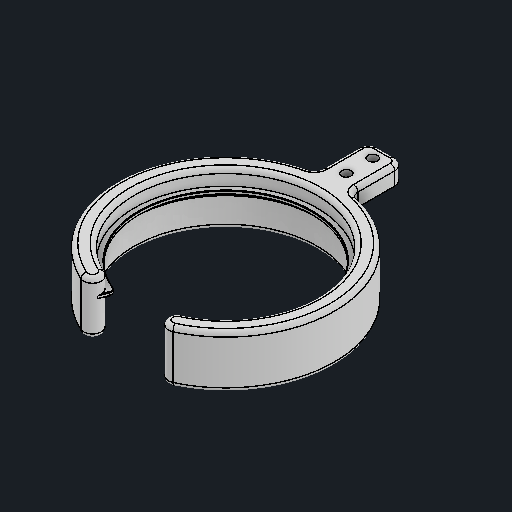
# Autodesk Inventor part: Can Clip
Saved by Autodesk Inventor 2026.2 (Build 302298000, 298)
## iProperties
Created: 2026-06-30
Part Number: Can Clip
Material: Generic
Document SubType Name: Modeling
Designer: JoshuaEah
Density: 1 g/cm^3
Appearance: Default
Author: JoshuaEah
Autodesk Inventor part; units mm, degrees
ref_plane "YZ Plane" through (0, 0, 0) normal (1, 0, 0) x (0, 1, 0)
ref_plane "XZ Plane" through (0, 0, 0) normal (0, 1, 0) x (-1, 0, 0)
ref_plane "XY Plane" through (0, 0, 0) normal (0, 0, 1) x (1, 0, 0)
sketch "Sketch1" plane through (0, 0, 0) normal (0, 1, 0) x (-1, 0, 0)
  circle A0 centre (0, 0) radius 33.02
  circle A1 centre (0, 0) radius 39.37
  line L0 (-10.642, 29.2385) -> (-13.4653, 36.9957)
  line L1 (0, 33.02) -> (0, -33.02)
  line L2 (10.642, 29.2385) -> (13.4653, 36.9957)
  line L3 (-6.35, -38.8545) -> (-6.35, -57.9045)
  line L4 (6.35, -38.8545) -> (6.35, -57.9045)
  line L5 (6.35, -57.9045) -> (-6.35, -57.9045)
  circle A2 centre (0, 0) radius 31.115
  circle A3 centre (0, -53.142) radius 1.5875
  line L6 (6.35, -48.3795) -> (-6.35, -48.3795) construction
  circle A4 centre (0, -43.617) radius 1.5875
  point P0 (13.4653, 36.9957)
  point P1 (11.2935, 31.0287)
  point P2 (-11.2935, 31.0287)
  point P3 (0, -31.115)
  point P4 (0, -48.3795)
  dimension "d11" = 62.23
  dimension "d0" = 66.04
  dimension "d1" = 6.35
  dimension "d2" = 20
  dimension "d5" = 12.7
  dimension "d6" = 19.05
  dimension "d22" = 3.175
  dimension "d24" = 4.7625
  constraints: 14 end point, 5 symmetric about line, 4 centre point, 4 midpoint, 4 point on circle, 2 coincident, 2 vertical, 1 horizontal, 1 line through centre, 1 vertical alignment, 4 other
  measures "d0" diameter of A0
  measures "d1" radial gap between concentric circles of A1 A0
  measures "d2" angle of L1 L0
  measures "d5" diameter of L3 L1
  measures "d6" distance of L3.start L3.end
  measures "d22" diameter of A3
  measures "d24" distance from line of A3.centre L6
extrude "Extrusion1" add sketch "Sketch1" along normal blind 6.35 contours A0 L2 A1 L0 | A1 L4 L5 L3 | A3 | A4 picked at (-15.3157, 33.7355)
extrude "Extrusion2" add sketch "Sketch1" against normal blind 12.7 contours A0 L2 A1 L0 picked at (-15.3157, 33.7355)
extrude "Extrusion3" add sketch "Sketch1" along normal mid plane 1.5875 contours L1 A2 L2 A0 | A0 L0 A2 L1 picked at (13.4667, 29.214) picked at (-13.3601, 29.285)
hole "Hole1" at (0, 0, -53.142) at (0, 0, -43.617) direction (0, 1, 0) diameter 3.4036 end through all start extended yes clearance for "Socket Head Cap Screw" size "M3" standard "Ansi Metric M Profile"
fillet "Fillet1" radius 3.175 10 edges at (-13.4653, -3.175, 36.9957) (13.4653, -3.175, 36.9957) (6.35, 3.175, -38.8545) (-6.35, 3.175, -38.8545) (-6.35, 3.175, -57.9045) (6.35, 3.175, -57.9045) (-11.2935, -6.7469, 31.0287) (11.2935, 3.5719, 31.0287) (11.2935, -6.7469, 31.0287) (-11.2935, 3.5719, 31.0287)
fillet "Fillet1" radius 1.5875 2 edges at (-10.642, 0, 29.2385) (10.642, 0, 29.2385)
chamfer "Chamfer1" distance 0.5292 angle 45 7 edges at (0, -0.7937, -31.115) (-11.2088, -0.7937, 29.5153) (-11.8126, -0.7937, 32.4548) (-11.2326, -0.7937, 30.8613) (11.2088, -0.7937, 29.5153) (11.2326, -0.7937, 30.8613) (11.8126, -0.7937, 32.4548)
chamfer "Chamfer2" distance 0.1984 angle 45 7 edges at (0, 0.7937, -31.115) (11.2088, 0.7937, 29.5153) (11.2326, 0.7937, 30.8613) (11.8126, 0.7937, 32.4548) (-11.2088, 0.7937, 29.5153) (-11.2326, 0.7937, 30.8613) (-11.8126, 0.7937, 32.4548)
fillet "Fillet2" radius 1.5875 12 edges at (39.1509, 6.35, -4.1478) (-39.1509, 6.35, -4.1478) (7.0413, 6.35, -39.4872) (6.35, 6.35, -48.0973) (5.4201, 6.35, -56.9746) (0, 6.35, -57.9045) (-5.4201, 6.35, -56.9746) (-6.35, 6.35, -48.0973) (-7.0413, 6.35, -39.4872) (0, 6.35, -33.02) (0, -12.7, -33.02) (0, -12.7, -39.37)
fillet "Fillet5" radius 1.3589 3 edges at (-12.8569, -0.7937, 30.7858) (12.8569, -0.7937, 30.7858) (0, -0.7937, -33.02)
equation "\"d24\" = 0.25 * d6"
body "Solid1"
